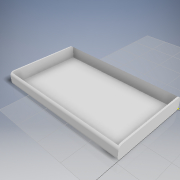
# Autodesk Inventor part: Raspberry Pi Phone Test
Saved by Autodesk Inventor 2018 (Build 220112000, 112)
## iProperties
Created: 2017-05-30
Part Number: Raspberry Pi Phone Test
Material: Generic
Document SubType Name: Modeling
Designer: Rishi
Density: 1 g/cm^3
Appearance: Default
Author: Rishi
Autodesk Inventor part; units mm, degrees
ref_plane "YZ Plane" through (0, 0, 0) normal (1, 0, 0) x (0, 1, 0)
ref_plane "XZ Plane" through (0, 0, 0) normal (0, 1, 0) x (-1, 0, 0)
ref_plane "XY Plane" through (0, 0, 0) normal (0, 0, 1) x (1, 0, 0)
sketch "Sketch1" plane through (0, 0, 0) normal (0, 1, 0) x (-1, 0, 0)
  line L0 (0, 0) -> (125, 0)
  line L1 (125, 0) -> (125, 75)
  line L2 (125, 75) -> (0, 75)
  line L3 (0, 75) -> (0, 0)
  dimension "d0" = 125
  dimension "d1" = 75
  constraints: 8 end point, 2 parallel, 1 horizontal, 1 perpendicular
  measures "d0" distance of L1.end L2.end
  measures "d1" distance of L0.end L1.end
extrude "Extrusion1" add sketch "Sketch1" along normal blind 1
sketch "Sketch2" plane through (0, 1, 0) normal (0, 1, 0) x (1, 0, 0)
  point P0 (0, 0)
sketch "Sketch3" plane through (0, 1, 0) normal (0, 1, 0) x (1, 0, 0)
  point P0 (0, 0)
sketch "Sketch4" plane through (0, 1, 0) normal (0, 1, 0) x (1, 0, 0)
  line L0 (-125, -75) -> (0, -75) projected
  line L1 (-125, -75) -> (0, -75)
  line L2 (0, -75) -> (0, 0)
  line L3 (0, 0) -> (-125, 0)
  line L4 (-125, 0) -> (-125, -75)
  line L5 (-123.5, -73.5) -> (-1.5, -73.5)
  line L6 (-1.5, -73.5) -> (-1.5, -1.5)
  line L7 (-1.5, -1.5) -> (-123.5, -1.5)
  line L8 (-123.5, -1.5) -> (-123.5, -73.5)
  dimension "d4" = 1.5
  dimension "d5" = 1.5
  dimension "d6" = 122
  dimension "d7" = 72
  constraints: 16 end point, 4 parallel, 2 horizontal, 2 perpendicular
  measures "d4" distance between parallel lines of L3 L7
  measures "d5" distance between parallel lines of L8 L4
  measures "d6" distance of L5.start L5.end
  measures "d7" distance of L7.end L5.start
extrude "Extrusion2" add sketch "Sketch4" along normal blind 13
fillet "Fillet1" radius 4 1 edges at (-62.5, 14, 75)
fillet "Fillet2" radius 4 1 edges at (-62.5, 14, 0)
fillet "Fillet3" radius 4 1 edges at (-62.5, 0, 75)
fillet "Fillet4" radius 4 1 edges at (-62.5, 0, 0)
body "Solid1"
